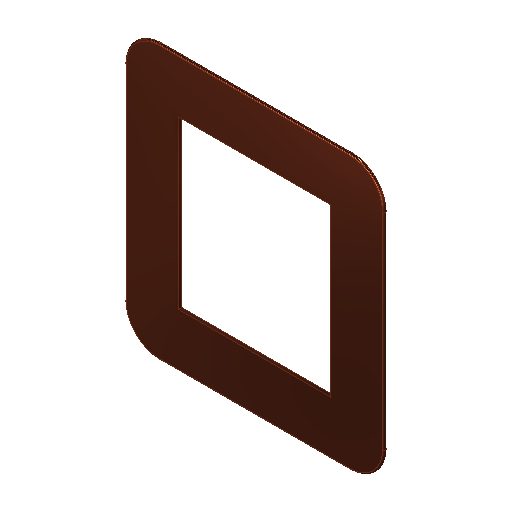
# Autodesk Inventor part: COTS_GENERIC_Transformer_Electromagnet_Coil_Layer
Saved by Autodesk Inventor 2026.1 (Build 301233000, 233)
## iProperties
Created: 2018-05-26
Part Number: COTS_GENERIC_Transformer_Electromagnet_Coil_Layer
Material: Copper
Document SubType Name: Modeling
Designer: Andrzej
Density: 8.94 g/cm^3
Appearance: Copper - Polished
Author: Andrzej
Autodesk Inventor part; units mm, degrees
ref_plane "YZ Plane" through (0, 0, 0) normal (1, 0, 0) x (0, 1, 0)
ref_plane "XZ Plane" through (0, 0, 0) normal (0, 1, 0) x (-1, 0, 0)
ref_plane "XY Plane" through (0, 0, 0) normal (0, 0, 1) x (1, 0, 0)
sketch "Sketch1" plane through (0, 0, 0) normal (0, 0, 1) x (1, 0, 0)
  line L0 (-6.5, 7.175) -> (6.5, 7.175)
  line L1 (6.5, 7.175) -> (6.5, -7.175)
  line L2 (6.5, -7.175) -> (-6.5, -7.175)
  line L3 (-6.5, -7.175) -> (-6.5, 7.175)
  line L4 (8.8, 12.475) -> (-8.8, 12.475)
  line L5 (-11.8, 9.475) -> (-11.8, -9.475)
  line L6 (-8.8, -12.475) -> (8.8, -12.475)
  line L7 (11.8, -9.475) -> (11.8, 9.475)
  arc A0 (-8.8, 12.475) -> (-11.8, 9.475) centre (-8.8, 9.475) ccw
  arc A1 (11.8, 9.475) -> (8.8, 12.475) centre (8.8, 9.475) ccw
  arc A2 (8.8, -12.475) -> (11.8, -9.475) centre (8.8, -9.475) ccw
  arc A3 (-11.8, -9.475) -> (-8.8, -12.475) centre (-8.8, -9.475) ccw
  line L8 (7, 7.675) -> (-7, 7.675)
  line L9 (-7, 7.675) -> (-7, -7.675)
  line L10 (-7, -7.675) -> (7, -7.675)
  line L11 (7, -7.675) -> (7, 7.675)
  point P0 (0, 0)
  dimension "d0" = 13
  dimension "d1" = 14.35
  dimension "d3" = 3
  dimension "d4" = 7.175
  dimension "d5" = 6.5
  dimension "d11" = 0.5
  dimension "d12" = 24.95
  dimension "d13" = 23.6
  constraints: 24 end point, 8 point on circle, 8 tangent, 6 parallel, 4 centre point, 3 equal radius, 3 perpendicular, 1 horizontal, 6 other
  measures "d0" distance of L1.end L2.end
  measures "d1" distance of L0.end L1.end
  measures "d3" radius of A0
  measures "d4" distance from line of point (0, 0) L0
  measures "d5" distance from line of L3 point (0, 0)
  measures "d11" distance between parallel lines of L0 L8
  measures "d12" distance between parallel lines of L4 L6
  measures "d13" distance between parallel lines of L7 L5
sketch "Sketch2" plane through (0, 0, 0) normal (0, 1, 0) x (-1, 0, 0)
  circle A0 centre (-11.8, 0) radius 0.15
  point P0 (0, 0)
  dimension "d6" = 0.3
  constraints: 1 centre point, 1 coincident
  measures "d6" diameter of A0
sweep "Sweep1" add profiles "Sketch2" path "Sketch1" path curves L5 A0 L4 A1 L7 A2 L6 A3
extrude "Extrusion1" add sketch "Sketch1" along normal mid plane 0.3 contours A1 L7 A2 L6 A3 L5 A0 L4
equation "\"d4\" = 0.5 * d1"
equation "\"d5\" = 0.5 * d0"
body "Solid1"
